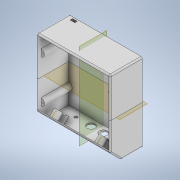
# Autodesk Inventor part: mávač_krabička
Saved by Autodesk Inventor 2022 (Build 260153000, 153)
## iProperties
Created: 2022-06-10
Part Number: mávač_krabička
Material: Generic
Document SubType Name: Modeling
Designer: Ruslana Zubareva
Density: 1 g/cm^3
Appearance: Default
Author: Ruslana Zubareva
Autodesk Inventor part; units mm, degrees
ref_plane "YZ Plane" through (0, 0, 0) normal (1, 0, 0) x (0, 1, 0)
ref_plane "XZ Plane" through (0, 0, 0) normal (0, 1, 0) x (-1, 0, 0)
ref_plane "XY Plane" through (0, 0, 0) normal (0, 0, 1) x (1, 0, 0)
sketch "Sketch1" plane through (0, 0, 0) normal (0, 0, 1) x (1, 0, 0)
  line L0 (0, 0) -> (150, 0)
  line L1 (150, 0) -> (150, -160)
  line L2 (150, -160) -> (0, -160)
  line L3 (0, -160) -> (0, 0)
  dimension "d0" = 150
  dimension "d1" = 160
  constraints: 8 end point, 2 parallel, 1 horizontal, 1 perpendicular
  measures "d0" distance of L1.end L2.end
  measures "d1" distance of L0.end L1.end
extrude "Extrusion1" add sketch "Sketch1" along normal blind 65
chamfer "Chamfer1" distance 25 angle 45 1 edges at (75, -160, 65)
shell "Shell1" thickness 3 outward yes removed faces 1 at (50, -45, 65)
fillet "Fillet1" radius 3 7 edges at (153, 3, 31) (-3, 3, 31) (-3, -151.1213, 53.1213) (153, -151.1213, 53.1213) (-3, -163, 19.1213) (153, -163, 19.1213) (75, -163, 41.2426)
fillet "Fillet2" radius 3 8 edges at (-2.1213, -138, 65) (75, -139.2426, 65) (152.1213, -138, 65) (153, -67.5, 65) (152.1213, 2.1213, 65) (75, 3, 65) (-2.1213, 2.1213, 65) (-3, -67.5, 65)
sketch "Sketch3" plane through (0, -162.1213, 42.1213) normal (0, -0.7071068, 0.7071068) x (1, 0, 0)
  line L0 (0, 35.3553) -> (0, 130.8148) projected
  line L1 (0, -28.2843) -> (0, 0) projected
  circle A0 centre (75, 16.6122) radius 7.5
  line L2 (0, 0) -> (0, 31.1127) projected
  line L3 (67.5, 16.6122) -> (27.5, 16.6122)
  circle A1 centre (27.5, 16.6122) radius 6.6
  line L4 (82.5, 16.6122) -> (122.5, 16.6122)
  circle A2 centre (122.5, 16.6122) radius 6.6
  point P0 (0, 84.8528)
  dimension "d12" = 15
  dimension "d13" = 75
  dimension "d18" = 40
  dimension "d19" = 13.2
  dimension "d20" = 40
  dimension "d21" = 13.2
  constraints: 4 end point, 3 centre point, 2 coincident, 2 point on circle, 2 point on line, 1 horizontal
  measures "d12" diameter of A0
  measures "d13" distance from line of L2 A0.centre
  measures "d18" distance of L3.start L3.end
  measures "d19" diameter of A1
  measures "d20" distance of L4.start L4.end
  measures "d21" diameter of A2
extrude "Extrusion2" cut sketch "Sketch3" against normal blind 10 contours A0
extrude "Extrusion3" cut sketch "Sketch3" against normal blind 10 contours A1 | A2
sketch "Sketch4" plane through (0, -163, -3) normal (0, -1, 0) x (1, 0, 0)
  line L0 (0, 43) -> (150, 43)
  line L1 (0, 43) -> (150, 43) projected
  line L2 (75, 43) -> (75, 0)
  circle A0 centre (30, 17.5) radius 3.25
  line L3 (150, 43) -> (150, 0) projected
  line L4 (0, 43) -> (150, 43) projected
  line L5 (0, 0) -> (0, 43) projected
  line L6 (0, 0) -> (150, 0) projected
  line L7 (0, 43) -> (150, 43) projected
  circle A1 centre (120, 17.5) radius 3.25
  dimension "d27" = 6.5
  dimension "d68" = 30
  dimension "d69" = 17.5
  constraints: 4 end point, 2 centre point, 1 midpoint, 1 symmetric about line, 1 vertical, 1 other
  measures "d27" diameter of A0
  measures "d68" distance from line of L5 A0.centre
  measures "d69" distance from line of L6 A0.centre
extrude "Extrusion4" cut sketch "Sketch4" against normal blind 10 contours A0 | A1
sketch "Sketch5" plane through (0, -163, -3) normal (0, -1, 0) x (1, 0, 0)
  line L0 (0, 43) -> (150, 43) projected
  line L1 (75, 43) -> (75, 3)
  line L2 (150, 3) -> (0, 3) projected
  line L3 (62, 17.5) -> (88, 17.5)
  circle A0 centre (88, 17.5) radius 8
  circle A1 centre (62, 17.5) radius 8
  circle A2 centre (120, 17.5) radius 3.25 projected
  circle A3 centre (30, 17.5) radius 3.25 projected
  dimension "d31" = 26
  dimension "d32" = 16
  dimension "d33" = 16
  dimension "d71" = 13
  constraints: 4 end point, 2 centre point, 2 coincident, 2 midpoint, 1 horizontal, 1 horizontal alignment
  measures "d31" distance of L3.start L3.end
  measures "d32" diameter of A0
  measures "d33" diameter of A1
  measures "d71" distance from line of L1 L3.start
extrude "Extrusion5" cut sketch "Sketch5" against normal blind 10 contours A0 | A1
sketch "Sketch6" plane through (0, 3, -3) normal (0, 1, 0) x (1, 0, 0)
  line L0 (150, -3) -> (0, -3) projected
  line L1 (8.7404, -3.5) -> (18.7404, -3.5)
  line L2 (18.7404, -3.5) -> (18.7404, -8.5)
  line L3 (18.7404, -8.5) -> (8.7404, -8.5)
  line L4 (8.7404, -8.5) -> (8.7404, -3.5)
  dimension "d36" = 10
  dimension "d37" = 5
  dimension "d49" = 0.5
  constraints: 8 end point, 2 parallel, 1 horizontal, 1 perpendicular
  measures "d36" distance of L2.end L3.end
  measures "d37" distance of L1.end L2.end
  measures "d49" distance between parallel lines of L0 L1
extrude "Extrusion6" cut sketch "Sketch6" against normal blind 10
sketch "Sketch10" plane through (0, 0, 0) normal (0, -1, 0) x (1, 0, 0)
  line L0 (0, 0) -> (0, 65) projected
  line L1 (3.7404, 12.4098) -> (43.7404, 12.4098)
  line L2 (43.7404, 12.4098) -> (43.7404, 0)
  line L3 (43.7404, 0) -> (3.7404, 0)
  line L4 (3.7404, 0) -> (3.7404, 12.4098)
  line L5 (8.7404, 5.5) -> (8.7404, 0.5) projected
  constraints: 8 end point, 2 parallel, 1 horizontal, 1 perpendicular
extrude "Extrusion8" cut sketch "Sketch10" against normal blind 2
sketch "Sketch11" plane through (0, -160, 0) normal (0, 0, 1) x (1, 0, 0)
  line L0 (0, 160) -> (0, 0) projected
  circle A0 centre (0, 125) radius 7.5
  line L1 (150, 163) -> (0, 163) projected
  circle A1 centre (3.5, 125) radius 1.5
  point P0 (0, 132.5)
  point P1 (0, 117.5)
  dimension "d52" = 15
  dimension "d53" = 38
  dimension "d54" = 3
  dimension "d55" = 3.5
  dimension "d56" = 38
  constraints: 2 centre point, 1 point on line
  measures "d52" diameter of A0
  measures "d53" distance from line of L1 A0.centre
  measures "d54" diameter of A1
  measures "d55" distance of A0.centre A1.centre
  measures "d56" distance from line of A1.centre L1
extrude "Extrusion9" add sketch "Sketch11" along normal blind 58 contours A0 L0 picked at (0.6667, 125)
sketch "Sketch12" plane through (3.5, -35, 0) normal (0, 0, 1) x (1, 0, 0)
  point P0 (-3.5, 35)
ref_plane "Work Plane2" through (75, -160, -3) normal (-1, 0, 0) x (0, 0, 1)
mirror "Mirror1" about plane through (75, -160, -3) normal (-1, 0, 0) of "Extrusion9"
ref_plane "Work Plane3" through (0, -80, -3) normal (0, 1, 0) x (1, 0, 0)
mirror "Mirror2" about plane through (0, -80, -3) normal (0, 1, 0) of "Extrusion9", "Mirror1"
sketch "Sketch13" plane through (0, -163, -3) normal (0, -1, 0) x (1, 0, 0)
  circle A0 centre (62, 17.5) radius 8 projected
  circle A1 centre (62, 17.5) radius 8.3
  circle A2 centre (88, 17.5) radius 8 projected
  circle A3 centre (88, 17.5) radius 8.3
  point P0 (0, 3)
  dimension "d59" = 16.6
  dimension "d60" = 16.6
  constraints: 2 centre point, 2 coincident
  measures "d59" diameter of A1
  measures "d60" diameter of A3
extrude "Extrusion10" cut sketch "Sketch13" against normal blind 12.9
sketch "Sketch14" plane through (0, -162.1213, 42.1213) normal (0, -0.7071068, 0.7071068) x (1, 0, 0)
  circle A0 centre (27.5, 16.6122) radius 6.6 projected
  circle A1 centre (27.5, 16.6122) radius 6.25
  circle A2 centre (122.5, 16.6122) radius 6.6 projected
  circle A3 centre (122.5, 16.6122) radius 6.25
  circle A4 centre (75, 16.6122) radius 7.5 projected
  circle A5 centre (75, 16.6122) radius 7.7
  point P0 (0, 84.8528)
  dimension "d63" = 12.5
  dimension "d64" = 12.5
  dimension "d65" = 15.4
  constraints: 3 centre point, 3 coincident
  measures "d63" diameter of A1
  measures "d64" diameter of A3
  measures "d65" diameter of A5
extrude "Extrusion11" cut sketch "Sketch14" against normal blind 20.85 contours A1 | A3 | A5
sketch "Sketch16" plane through (150, -160, 40) normal (0, 0.7071068, -0.7071068) x (-1, 0, 0)
  circle A0 centre (122.5, 16.6122) radius 6.25 projected
  line L0 (19, 6.6122) -> (36, 6.6122)
  line L1 (36, 6.6122) -> (36, 26.6122)
  line L2 (36, 26.6122) -> (19, 26.6122)
  line L3 (19, 26.6122) -> (19, 6.6122)
  line L4 (19, 6.6122) -> (36, 26.6122) construction
  line L5 (36, 6.6122) -> (19, 26.6122) construction
  circle A1 centre (27.5, 16.6122) radius 7.25
  line L6 (19, 24.6122) -> (36, 24.6122)
  line L7 (21.25, 16.6122) -> (33.75, 16.6122) construction
  line L8 (19, 8.6122) -> (36, 8.6122)
  circle A2 centre (27.5, 16.6122) radius 6.6 projected
  point P0 (150, 84.8528)
  point P1 (19, 8.6122)
  point P2 (36, 8.6122)
  dimension "d72" = 17
  dimension "d73" = 20
  dimension "d74" = 14.5
  dimension "d75" = 2
  constraints: 18 end point, 3 midpoint, 3 perpendicular, 2 parallel, 2 point on line, 2 symmetric about line, 1 centre point, 1 coincident, 1 concentric, 1 horizontal, 1 horizontal alignment
  measures "d72" distance of L2.end L1.end
  measures "d73" distance of L1.end L0.end
  measures "d74" diameter of A1
  measures "d75" distance between parallel lines of L2 L6
extrude "Extrusion12" add sketch "Sketch16" along normal blind 14 contours L3 L8 L1 L0 | L3 L2 L1 L6
sketch "Sketch17" plane through (114, -153.9103, 46.0897) normal (0, 0.7071068, 0.7071068) x (1, 0, 0)
  line L0 (17, 14) -> (0, 14) projected
  line L1 (17, 14) -> (0, 14)
  line L2 (0, 14) -> (0, 12)
  line L3 (0, 12) -> (17, 12)
  line L4 (17, 12) -> (17, 14)
  point P0 (-114, 141.4214)
  point P1 (0, 14)
  dimension "d78" = 17
  dimension "d79" = 2
  constraints: 8 end point, 2 parallel, 1 horizontal, 1 perpendicular
  measures "d78" distance of L3.end L2.end
  measures "d79" distance of L2.end L1.end
extrude "Extrusion13" add sketch "Sketch17" along normal up to surface (16 mm away)
sketch "Sketch18" plane through (114, -155.3245, 44.6755) normal (-1, 0, 0) x (0, -0.7071068, 0.7071068)
  line L0 (-12, 2) -> (-12, 18) projected
  line L1 (-12, 18) -> (-14, 18)
  line L2 (-14, 18) -> (-14, 2)
  line L3 (-14, 2) -> (-12, 2)
  line L4 (-12, 2) -> (-12, 18)
  point P0 (-141.4214, 78.2407)
  point P1 (-12, 2)
  dimension "d82" = 2
  dimension "d83" = 16
  constraints: 8 end point, 2 parallel, 1 horizontal, 1 perpendicular
  measures "d82" distance of L3.end L2.end
  measures "d83" distance of L2.end L1.end
extrude "Extrusion14" cut sketch "Sketch18" against normal blind 4
ref_plane "Work Plane4" through (122.5, -142.5966, 57.4034) normal (-1, 0, 0) x (0, -0.7071068, 0.7071068)
mirror "Mirror3" about plane through (122.5, -142.5966, 57.4034) normal (-1, 0, 0) of "Extrusion14"
mirror "Mirror4" about plane through (75, -160, -3) normal (-1, 0, 0) of "Extrusion12", "Extrusion13", "Extrusion14", "Mirror3"
split body "Split1" result two bodies by plane through (0, -80, -3) normal (0, 1, 0) first body at (100, -52.3333, -2.5)
ref_plane "Work Plane5" through (27.5, -142.5966, 57.4034) normal (-1, 0, 0) x (0, -0.7071068, 0.7071068)
body "Solid2"
body "Solid3"
